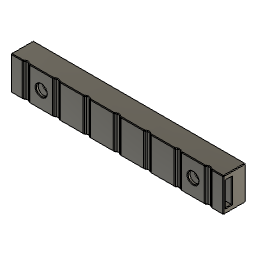
model (Autodesk Fusion 360 design; units mm, degrees)
Autodesk Fusion 360 part; units mm, degrees
note: some values were not read from the file. Set by a fixed rule: which face or edge a step refers to.
sketch "Sketch1" plane through (0, 0, 0) normal (0, 0, 1) x (1, 0, 0)
  line L0 (0, 0) -> (500, 0)
  line L1 (500, 0) -> (500, 12)
  line L2 (500, 12) -> (0, 12)
  line L3 (0, 12) -> (0, 0)
  line L4 (9.9019, 0) -> (12.5, 1.5)
  line L5 (12.5, 1.5) -> (15.0981, 0)
  circle A0 centre (12.5, -3.1188) radius 4 construction
  line L6 (34.9019, 0) -> (37.5, 1.5)
  line L7 (37.5, 1.5) -> (40.0981, 0)
  line L8 (59.9019, 0) -> (62.5, 1.5)
  line L9 (62.5, 1.5) -> (65.0981, 0)
  line L10 (84.9019, 0) -> (87.5, 1.5)
  line L11 (87.5, 1.5) -> (90.0981, 0)
  line L12 (109.9019, 0) -> (112.5, 1.5)
  line L13 (112.5, 1.5) -> (115.0981, 0)
  line L14 (134.9019, 0) -> (137.5, 1.5)
  line L15 (137.5, 1.5) -> (140.0981, 0)
  line L16 (159.9019, 0) -> (162.5, 1.5)
  line L17 (162.5, 1.5) -> (165.0981, 0)
  line L18 (184.9019, 0) -> (187.5, 1.5)
  line L19 (187.5, 1.5) -> (190.0981, 0)
  line L20 (209.9019, 0) -> (212.5, 1.5)
  line L21 (212.5, 1.5) -> (215.0981, 0)
  line L22 (234.9019, 0) -> (237.5, 1.5)
  line L23 (237.5, 1.5) -> (240.0981, 0)
  line L24 (259.9019, 0) -> (262.5, 1.5)
  line L25 (262.5, 1.5) -> (265.0981, 0)
  line L26 (284.9019, 0) -> (287.5, 1.5)
  line L27 (287.5, 1.5) -> (290.0981, 0)
  line L28 (309.9019, 0) -> (312.5, 1.5)
  line L29 (312.5, 1.5) -> (315.0981, 0)
  line L30 (334.9019, 0) -> (337.5, 1.5)
  line L31 (337.5, 1.5) -> (340.0981, 0)
  line L32 (359.9019, 0) -> (362.5, 1.5)
  line L33 (362.5, 1.5) -> (365.0981, 0)
  line L34 (384.9019, 0) -> (387.5, 1.5)
  line L35 (387.5, 1.5) -> (390.0981, 0)
  line L36 (409.9019, 0) -> (412.5, 1.5)
  line L37 (412.5, 1.5) -> (415.0981, 0)
  line L38 (434.9019, 0) -> (437.5, 1.5)
  line L39 (437.5, 1.5) -> (440.0981, 0)
  line L40 (459.9019, 0) -> (462.5, 1.5)
  line L41 (462.5, 1.5) -> (465.0981, 0)
  line L42 (484.9019, 0) -> (487.5, 1.5)
  line L43 (487.5, 1.5) -> (490.0981, 0)
  line L44 (0, 2) -> (500, 2)
  line L45 (175, 12) -> (175, 0)
  dimension "d1" = 500
  dimension "d3" = 12.5
  dimension "d5" = 8
  dimension "d8" = 25
  dimension "d9" = 0
  dimension "d10" = 10
  dimension "d11" = 2
  dimension "d12" = 175
  dimension "d14" = 120
  dimension "d16" = 0.5
  constraint horizontal L0
  constraint vertical L1
  constraint horizontal L2
  constraint vertical L3
  constraint coincident L0.start L3.end
  constraint coincident L0 L4.start
  constraint coincident L0 L5.end
  constraint equal L4 L5
  constraint tangent L4 A0
  constraint coincident L3 L44.start
  constraint horizontal L44
  constraint coincident L2 L45.start
  constraint coincident L0 L45.end
  constraint vertical L45
  constraint tangent L5 A0
  measures "d1" distance of L0.start L0.end
  measures "d3" horizontal distance of L0.start L4.end
  measures "d5" diameter of A0
  measures "d10" distance of L2.end L44.start
  measures "d11" distance of L0.start L44.start
  measures "d12" distance of L2.end L45.start
  measures "d14" angle of L4 L5
  measures "d16" vertical distance of L4.end L44.start
extrude "Extrude1" add sketch "Sketch1" along normal blind 4 contours L0 L3 L4 L5 L6 L7 L8 L9 L10 L11 L12 L13 L14 L15 L16 L17 L44 L45 | L2 L3 L44 L45
extrude "Extrude2" add sketch "Sketch1" along normal blind 19.75 from surface at 4 contours L0 L3 L4 L5 L6 L7 L8 L9 L10 L11 L12 L13 L14 L15 L16 L17 L44 L45
extrude "Extrude3" add sketch "Sketch1" along normal blind 4 from surface at 23.75 contours L0 L3 L4 L5 L6 L7 L8 L9 L10 L11 L12 L13 L14 L15 L16 L17 L44 L45 | L2 L3 L44 L45
sketch "Sketch2" plane through (0, 12, 0) normal (0, 1, 0) x (-1, 0, 0)
  line L0 (-175, 23.75) -> (0, 23.75)
  line L1 (0, 23.75) -> (0, 27.75)
  line L2 (0, 27.75) -> (-175, 27.75)
  line L3 (-175, 27.75) -> (-175, 23.75)
  line L4 (-175, 27.75) -> (0, 27.75)
  line L5 (0, 27.75) -> (0, 0)
  line L6 (0, 0) -> (-175, 0)
  line L7 (-175, 0) -> (-175, 27.75)
  line L8 (-15.0981, 0) -> (-34.9019, 0)
  line L9 (-34.9019, 0) -> (-34.9019, 27.75)
  line L10 (-34.9019, 27.75) -> (-15.0981, 27.75)
  line L11 (-15.0981, 27.75) -> (-15.0981, 0)
  line L12 (-40.0981, 0) -> (-59.9019, 0)
  line L13 (-59.9019, 0) -> (-59.9019, 27.75)
  line L14 (-59.9019, 27.75) -> (-40.0981, 27.75)
  line L15 (-40.0981, 27.75) -> (-40.0981, 0)
  line L16 (-65.0981, 0) -> (-84.9019, 0)
  line L17 (-84.9019, 0) -> (-84.9019, 27.75)
  line L18 (-84.9019, 27.75) -> (-65.0981, 27.75)
  line L19 (-65.0981, 27.75) -> (-65.0981, 0)
  line L20 (-90.0981, 0) -> (-109.9019, 0)
  line L21 (-109.9019, 0) -> (-109.9019, 27.75)
  line L22 (-109.9019, 27.75) -> (-90.0981, 27.75)
  line L23 (-90.0981, 27.75) -> (-90.0981, 0)
  line L24 (-115.0981, 0) -> (-134.9019, 0)
  line L25 (-134.9019, 0) -> (-134.9019, 27.75)
  line L26 (-134.9019, 27.75) -> (-115.0981, 27.75)
  line L27 (-115.0981, 27.75) -> (-115.0981, 0)
  line L28 (-140.0981, 0) -> (-159.9019, 0)
  line L29 (-159.9019, 0) -> (-159.9019, 27.75)
  line L30 (-159.9019, 27.75) -> (-140.0981, 27.75)
  line L31 (-140.0981, 27.75) -> (-140.0981, 0)
  line L32 (-165.0981, 0) -> (-175, 0)
  line L33 (-175, 0) -> (-175, 27.75)
  line L34 (-175, 27.75) -> (-165.0981, 27.75)
  line L35 (-165.0981, 27.75) -> (-165.0981, 0)
  line L36 (0, 0) -> (-9.9019, 0)
  line L37 (-9.9019, 0) -> (-9.9019, 27.75)
  line L38 (-9.9019, 27.75) -> (0, 27.75)
  line L39 (0, 27.75) -> (0, 0)
  circle A0 centre (-150, 13.875) radius 2.25
  circle A1 centre (-25, 13.875) radius 2.25
  line L40 (-34.9019, 13.875) -> (-15.0981, 13.875) construction
  line L41 (-159.9019, 13.875) -> (-140.0981, 13.875) construction
  dimension "d27" = 4.5
  constraint horizontal L4
  constraint vertical L5
  constraint horizontal L6
  constraint vertical L7
  constraint coincident L5.end L6.start
  constraint coincident L2.end L3.start
  constraint midpoint L9 L40.start
  constraint midpoint L11 L40.end
  constraint midpoint L29 L41.start
  constraint midpoint L31 L41.end
  constraint midpoint A0.centre L41
  constraint midpoint A1.centre L40
  constraint equal A0 A1
  measures "d27" diameter of A1
extrude "Extrude4" add sketch "Sketch2" 1 faces at (116.6667, 12, 25.0833) along normal blind 6
extrude "Extrude5" cut sketch "Sketch2" against normal up to surface (12 mm away) contours A0 | A1
chamfer "Chamfer1" distance 4 angle 45 2 edges at (27.0977, 12, 14.6886) (152.0977, 12, 14.6886)
move_face "OffsetFaces1" offset -2.25 2 faces at (149.6093, 1.3333, 16.0908) (22.7612, 1.3333, 13.651)
extrude "Extrude6" add 1 faces at (168.75, 12, 13.875) along direction (0, -1, 0) blind 5
fillet "Fillet1" radius 2 21 edges at (12.5, 1.5, 13.875) (37.5, 1.5, 13.875) (62.5, 1.5, 13.875) (87.5, 1.5, 13.875) (112.5, 1.5, 13.875) (137.5, 1.5, 13.875) (162.5, 1.5, 13.875) (9.9019, 0, 13.875) (15.0981, 0, 13.875) (34.9019, 0, 13.875) (40.0981, 0, 13.875) (59.9019, 0, 13.875) (65.0981, 0, 13.875) (84.9019, 0, 13.875) (90.0981, 0, 13.875) (109.9019, 0, 13.875) (115.0981, 0, 13.875) (134.9019, 0, 13.875) (140.0981, 0, 13.875) (159.9019, 0, 13.875) (165.0981, 0, 13.875)
chamfer "Chamfer2" distance 0.5 angle 45 102 edges at (4.683, 0, 27.75) (9.8837, 0.0681, 27.75) (10.933, 0.5953, 27.75) (12.5, 1.1906, 27.75) (14.067, 0.5953, 27.75) (15.1163, 0.0681, 27.75) (25, 0, 27.75) (34.8837, 0.0681, 27.75) (35.933, 0.5953, 27.75) (37.5, 1.1906, 27.75) (39.067, 0.5953, 27.75) (40.1163, 0.0681, 27.75) (50, 0, 27.75) (59.8837, 0.0681, 27.75) (60.933, 0.5953, 27.75) (62.5, 1.1906, 27.75) (64.067, 0.5953, 27.75) (65.1163, 0.0681, 27.75) (75, 0, 27.75) (84.8837, 0.0681, 27.75) (85.933, 0.5953, 27.75) (87.5, 1.1906, 27.75) (89.067, 0.5953, 27.75) (90.1163, 0.0681, 27.75) (100, 0, 27.75) (109.8837, 0.0681, 27.75) (110.933, 0.5953, 27.75) (112.5, 1.1906, 27.75) (114.067, 0.5953, 27.75) (115.1163, 0.0681, 27.75) (125, 0, 27.75) (134.8837, 0.0681, 27.75) (135.933, 0.5953, 27.75) (137.5, 1.1906, 27.75) (139.067, 0.5953, 27.75) (140.1163, 0.0681, 27.75) (150, 0, 27.75) (159.8837, 0.0681, 27.75) (160.933, 0.5953, 27.75) (162.5, 1.1906, 27.75) (164.067, 0.5953, 27.75) (165.1163, 0.0681, 27.75) (170.317, 0, 27.75) (4.683, 0, 0) (9.8837, 0.0681, 0) (10.933, 0.5953, 0) (12.5, 1.1906, 0) (14.067, 0.5953, 0) (15.1163, 0.0681, 0) (25, 0, 0) (34.8837, 0.0681, 0) (35.933, 0.5953, 0) (37.5, 1.1906, 0) (39.067, 0.5953, 0) (40.1163, 0.0681, 0) (50, 0, 0) (59.8837, 0.0681, 0) (60.933, 0.5953, 0) (62.5, 1.1906, 0) (64.067, 0.5953, 0) (65.1163, 0.0681, 0) (75, 0, 0) (84.8837, 0.0681, 0) (85.933, 0.5953, 0) (87.5, 1.1906, 0) (89.067, 0.5953, 0) (90.1163, 0.0681, 0) (100, 0, 0) (109.8837, 0.0681, 0) (110.933, 0.5953, 0) (112.5, 1.1906, 0) (114.067, 0.5953, 0) (115.1163, 0.0681, 0) (125, 0, 0) (134.8837, 0.0681, 0) (135.933, 0.5953, 0) (137.5, 1.1906, 0) (139.067, 0.5953, 0) (140.1163, 0.0681, 0) (150, 0, 0) (159.8837, 0.0681, 0) (160.933, 0.5953, 0) (162.5, 1.1906, 0) (164.067, 0.5953, 0) (165.1163, 0.0681, 0) (170.317, 0, 0) (0, 7, 13.875) (0, 4.5, 23.75) (0, 2, 13.875) (0, 4.5, 4) (175, 4.5, 23.75) (175, 2, 13.875) (175, 7, 13.875) (175, 4.5, 4) (0, 9, 27.75) (0, 0, 13.875) (0, 9, 0) (175, 9, 27.75) (175, 0, 13.875) (175, 9, 0) (154.1955, 0, 12.2477) (29.1955, 0, 12.2477)
equation "d1 = ( 25 * 20 ) * 1 mm"
equation "d3 = sp / 2"
equation "d12 = 7 * sp"
equation "sp = 25 mm"
